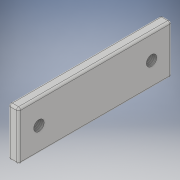
# Autodesk Inventor part: Clamp Plate
Saved by Autodesk Inventor 2019 (Build 230136000, 136)
## iProperties
Created: 2019-06-10
Part Number: Clamp Plate
Material: Generic
Document SubType Name: Modeling
Designer: Matthew XPS
Density: 1 g/cm^3
Appearance: Default
Author: Matthew XPS
Autodesk Inventor part; units mm, degrees
ref_plane "YZ Plane" through (0, 0, 0) normal (1, 0, 0) x (0, 1, 0)
ref_plane "XZ Plane" through (0, 0, 0) normal (0, 1, 0) x (-1, 0, 0)
ref_plane "XY Plane" through (0, 0, 0) normal (0, 0, 1) x (1, 0, 0)
sketch "Sketch1" plane through (0, 0, 0) normal (1, 0, 0) x (0, 1, 0)
  line L0 (-7, 22) -> (-7, -22)
  line L1 (-7, -22) -> (7, -22)
  line L2 (7, -22) -> (7, 22)
  line L3 (7, 22) -> (-7, 22)
  line L4 (-7, 22) -> (7, -22) construction
  line L5 (-7, -22) -> (7, 22) construction
  point P0 (0, 0)
  dimension "d0" = 44
  dimension "d1" = 14
  constraints: 12 end point, 2 midpoint, 2 parallel, 1 perpendicular, 1 vertical
  measures "d0" distance of L0.start L0.end
  measures "d1" distance of L1.end L0.end
extrude "Extrusion1" add sketch "Sketch1" along normal blind 3
sketch "Sketch2" plane through (3, 0, 0) normal (1, 0, 0) x (0, 0, -1)
  line L0 (0, 0) -> (16.154, 0)
  circle A0 centre (16.154, 0) radius 1.5
  dimension "d4" = 16.154
  dimension "d5" = 3
  constraints: 2 end point, 1 centre point, 1 coincident, 1 horizontal
  measures "d4" distance of L0.start L0.end
  measures "d5" diameter of A0
extrude "Extrusion2" cut sketch "Sketch2" against normal blind 3
thread "Thread1" size "M3x0.5" class "6H" standard "ANSI Metric M Profile" full length
mirror "Mirror1" about plane through (0, 0, 0) normal (0, 0, 1) of "Extrusion2"
fillet "Fillet1" radius 0.6 12 edges at (3, -7, 0) (0, -7, 0) (1.5, -7, -22) (3, 0, -22) (0, 0, -22) (1.5, 7, -22) (3, 7, 0) (0, 7, 0) (1.5, 7, 22) (3, 0, 22) (1.5, -7, 22) (0, 0, 22)
body "Solid1"
